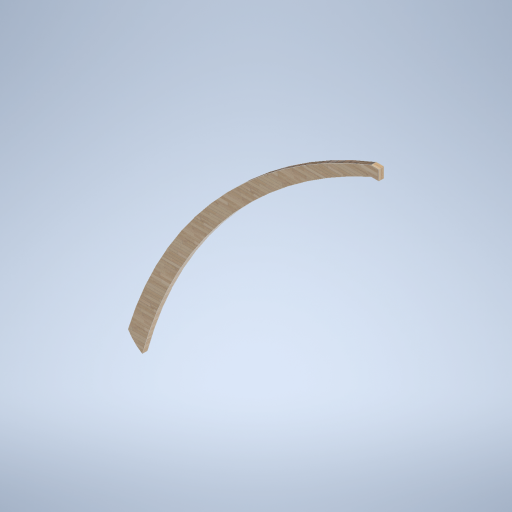
# Autodesk Inventor part: curve_beam_01
Saved by Autodesk Inventor 2024.2 (Build 282272000, 272)
## iProperties
Created: 2024-05-19
Part Number: curve_beam_01
Material: Wood (Maple)
Document SubType Name: Modeling
Designer: LOSTER_1
Density: 0.67 g/cm^3
Appearance: Natural Maple - Glossy Dark Tint
Author: LOSTER_1
Autodesk Inventor part; units mm, degrees
ref_plane "YZ Plane" through (0, 0, 0) normal (1, 0, 0) x (0, 1, 0)
ref_plane "XZ Plane" through (0, 0, 0) normal (0, 1, 0) x (-1, 0, 0)
ref_plane "XY Plane" through (0, 0, 0) normal (0, 0, 1) x (1, 0, 0)
sketch "Sketch1" plane through (0, 0, 0) normal (0, 0, 1) x (1, 0, 0)
  line L0 (4856.4349, 5392.3386) -> (4856.4349, 5192.3386)
  arc A0 (4706.4349, 5392.28) -> (-20.5961, 263.191) centre (7637.2096, -2051.5469) ccw
  ellipse E0 centre (665.286, 674.9746) end of major axis (665.286, -125.0254) minor radius 800 (-20.5961, 263.191) -> (256.6451, -12.7845) ccw
  arc A1 (4706.4349, 5192.3386) -> (256.6451, -12.7845) centre (7977.2775, -2108.4551) ccw
  line L1 (4706.4349, 5392.28) -> (4706.4349, 5392.3386)
  line L2 (4706.4349, 5392.3386) -> (4856.4349, 5392.3386)
  line L3 (4706.4349, 5192.3386) -> (4856.4349, 5192.3386)
  point P0 (0, 0)
  constraints: 8 end point, 4 point on circle, 2 centre point, 1 horizontal, 4 other
extrude "Extrusion1" add sketch "Sketch1" along normal blind 100
body "Solid1"
